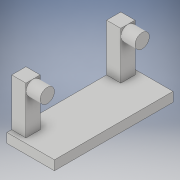
# Autodesk Inventor part: LaserMountTop
Saved by Autodesk Inventor 2019 (Build 230136000, 136)
## iProperties
Created: 2019-05-18
Part Number: LaserMountTop
Material: Generic
Document SubType Name: Modeling
Designer: Henry
Density: 1 g/cm^3
Appearance: Default
Author: Henry
Autodesk Inventor part; units mm, degrees
ref_plane "YZ Plane" through (0, 0, 0) normal (1, 0, 0) x (0, 1, 0)
ref_plane "XZ Plane" through (0, 0, 0) normal (0, 1, 0) x (-1, 0, 0)
ref_plane "XY Plane" through (0, 0, 0) normal (0, 0, 1) x (1, 0, 0)
sketch "Sketch1" plane through (0, 0, 0) normal (0, 1, 0) x (-1, 0, 0)
  line L0 (0, 0) -> (10, 0)
  line L1 (10, 0) -> (10, -25)
  line L2 (10, -25) -> (0, -25)
  line L3 (0, -25) -> (0, 0)
  dimension "d0" = 10
  dimension "d1" = 25
  constraints: 8 end point, 2 parallel, 1 horizontal, 1 perpendicular
  measures "d0" distance of L1.end L2.end
  measures "d1" distance of L0.end L1.end
extrude "Extrusion1" add sketch "Sketch1" along normal blind 2
sketch "Sketch2" plane through (0, 2, 0) normal (0, 1, 0) x (1, 0, 0)
  line L0 (-10, 0) -> (0, 0) projected
  line L1 (-10, 0) -> (-10, 1)
  line L2 (-10, 1) -> (-7, 1)
  line L3 (-7, 1) -> (-7, 4)
  line L4 (-7, 4) -> (-10, 4)
  line L5 (-10, 4) -> (-10, 1)
  line L6 (0, 25) -> (-10, 25) projected
  line L7 (-10, 25) -> (-10, 24)
  line L8 (-10, 24) -> (-7, 24)
  line L9 (-7, 24) -> (-7, 21)
  line L10 (-7, 21) -> (-10, 21)
  line L11 (-10, 21) -> (-10, 24)
  dimension "d4" = 1
  dimension "d5" = 3
  dimension "d6" = 3
  dimension "d7" = 1
  dimension "d8" = 3
  dimension "d9" = 3
  constraints: 20 end point, 4 parallel, 2 horizontal, 2 perpendicular, 2 vertical
  measures "d4" distance of L0.start L1.end
  measures "d5" distance of L4.end L3.end
  measures "d6" distance of L3.end L2.end
  measures "d7" distance of L6.end L7.end
  measures "d8" distance of L9.end L10.end
  measures "d9" distance of L8.end L9.end
extrude "Extrusion2" add sketch "Sketch2" along normal blind 10
sketch "Sketch3" plane through (-7, 2, -1) normal (1, 0, 0) x (0, 0, -1)
  line L0 (0, 0) -> (0, 10) projected
  line L1 (0, 10) -> (1.5, 10)
  line L2 (1.5, 10) -> (1.5, 8.5)
  line L3 (1.5, 8.5) -> (0, 8.5)
  line L4 (0, 8.5) -> (0, 10)
  line L5 (23, 10) -> (20, 10) projected
  line L6 (23, 10) -> (21.5, 10)
  line L7 (21.5, 10) -> (21.5, 8.5)
  line L8 (21.5, 8.5) -> (23, 8.5)
  line L9 (23, 8.5) -> (23, 10)
  circle A0 centre (1.5, 8.5) radius 1.5
  circle A1 centre (21.5, 8.5) radius 1.5
  point P0 (-1, -2)
  dimension "d12" = 1.5
  dimension "d13" = 1.5
  dimension "d14" = 1.5
  dimension "d15" = 1.5
  dimension "d16" = 3
  dimension "d17" = 3
  constraints: 16 end point, 4 parallel, 2 centre point, 2 coincident, 2 horizontal, 2 perpendicular
  measures "d12" distance of L2.end L3.end
  measures "d13" distance of L1.end L2.end
  measures "d14" distance of L8.end L7.end
  measures "d15" distance of L7.end L6.end
  measures "d16" diameter of A0
  measures "d17" diameter of A1
extrude "Extrusion3" add sketch "Sketch3" along normal blind 3 contours A0 L2 L3 | L3 L2 A0 | A1 L8 L7 | L7 L8 A1
body "Solid1"
